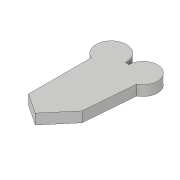
# Autodesk Inventor part: TestPart
Saved by Autodesk Inventor 2019 (Build 230136000, 136)
## iProperties
Created: 2019-09-22
Part Number: TestPart
Material: Generic
Document SubType Name: Modeling
Designer: Lord of Xy
Density: 1 g/cm^3
Appearance: Default
Author: Lord of Xy
Autodesk Inventor part; units mm, degrees
ref_plane "YZ Plane" through (0, 0, 0) normal (1, 0, 0) x (0, 1, 0)
ref_plane "XZ Plane" through (0, 0, 0) normal (0, 1, 0) x (-1, 0, 0)
ref_plane "XY Plane" through (0, 0, 0) normal (0, 0, 1) x (1, 0, 0)
sketch "Sketch1" plane through (0, 0, 0) normal (0, 1, 0) x (-1, 0, 0)
  arc A0 (0.6157, -1.2811) -> (5.8771, 1.956) centre (4.3727, -1.4931) ccw
  arc A1 (-5.4159, 1.956) -> (-0.2522, -1.2087) centre (-3.8039, -1.2087) ccw
  line L0 (5.8771, 1.956) -> (5.8771, 17.4195)
  line L1 (5.8771, 17.4195) -> (0.9243, 20.7257)
  line L2 (0.9243, 20.7257) -> (-4.3727, 14.4689)
  line L3 (-4.3727, 14.4689) -> (-5.4159, 1.956)
  line L4 (-0.2522, -1.2087) -> (0.6157, -1.2811)
  point P0 (0, 0)
  constraints: 10 end point, 4 point on circle, 2 centre point, 1 perpendicular, 1 vertical
extrude "Extrusion1" add sketch "Sketch1" along normal blind 2.54
body "Solid1"
